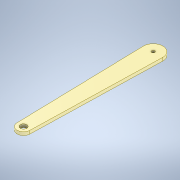
# Autodesk Inventor part: Canh_Tay_2
Saved by Autodesk Inventor 2022 (Build 260153000, 153)
## iProperties
Created: 2022-11-10
Part Number: Canh_Tay_2
Material: Nylon 6/6
Document SubType Name: Modeling
Designer: nguye
Density: 1.13 g/cm^3
Appearance: Nylon 6
Author: nguye
Autodesk Inventor part; units mm, degrees
ref_plane "YZ Plane" through (0, 0, 0) normal (1, 0, 0) x (0, 1, 0)
ref_plane "XZ Plane" through (0, 0, 0) normal (0, 1, 0) x (-1, 0, 0)
ref_plane "XY Plane" through (0, 0, 0) normal (0, 0, 1) x (1, 0, 0)
sketch "Sketch1" plane through (0, 0, 0) normal (0, 1, 0) x (-1, 0, 0)
  circle A0 centre (0, 0) radius 2.5
  circle A1 centre (0, 0) radius 15
  circle A2 centre (0, 200) radius 5
  circle A3 centre (0, 200) radius 10
  line L0 (9.9969, 200.25) -> (14.9953, 0.375)
  line L1 (-9.9969, 200.25) -> (-14.9953, 0.375)
  dimension "d0" = 5
  dimension "d1" = 30
  dimension "d2" = 10
  dimension "d3" = 200
  dimension "d4" = 20
  constraints: 4 centre point, 4 end point, 4 point on circle, 4 tangent, 3 coincident, 1 vertical alignment
  measures "d0" diameter of A0
  measures "d1" diameter of A1
  measures "d2" diameter of A2
  measures "d3" distance of point (0, 0) A2.centre
  measures "d4" diameter of A3
extrude "Extrusion1" add sketch "Sketch1" along normal blind 5
body "Solid1"
